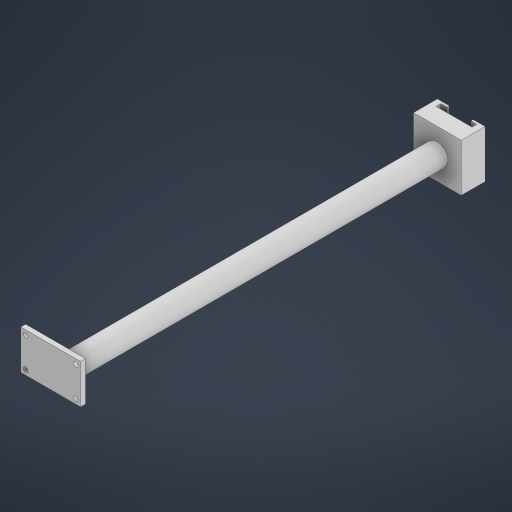
# Autodesk Inventor part: camera arm v1
Saved by Autodesk Inventor 2024 (Build 280153000, 153)
## iProperties
Created: 2023-06-18
Part Number: camera arm v1
Material: 일반
Document SubType Name: Modeling
Designer: 6gioc
Density: 1 g/cm^3
Appearance: 기본값
Author: 6gioc
## iProperties of the stored document camera arm v1_3D 인쇄.ipt
Created: 2023-06-20
Part Number: camera arm v1_3D 인쇄
Material: 일반
Document SubType Name: Modeling
Designer: 6gioc
Density: 1 g/cm^3
Appearance: 기본값
Author: 6gioc
Autodesk Inventor part; units mm, degrees
ref_plane "YZ Plane" through (0, 0, 0) normal (1, 0, 0) x (0, 1, 0)
ref_plane "XZ Plane" through (0, 0, 0) normal (0, 1, 0) x (-1, 0, 0)
ref_plane "XY Plane" through (0, 0, 0) normal (0, 0, 1) x (1, 0, 0)
sketch "스케치1" plane through (0, 0, 0) normal (0, 0, 1) x (1, 0, 0)
  line L0 (0, 0) -> (25, 0)
  line L1 (25, 0) -> (25, 16.5)
  line L2 (25, 16.5) -> (0, 16.5)
  line L3 (0, 16.5) -> (0, 0)
  circle A0 centre (23, 14.5) radius 1
  circle A1 centre (2, 14.5) radius 1
  circle A2 centre (2, 2) radius 1
  circle A3 centre (23, 2) radius 1
  circle A4 centre (12.5, 4.5) radius 4.5
  dimension "d0" = 25
  dimension "d1" = 16.5
  dimension "d2" = 2
  dimension "d3" = 2
  dimension "d4" = 2
  dimension "d5" = 2
  dimension "d6" = 2
  dimension "d7" = 2
  dimension "d8" = 2
  dimension "d9" = 2
  dimension "d10" = 2
  dimension "d11" = 2
  dimension "d12" = 2
  dimension "d13" = 2
  dimension "d14" = 12.5
  dimension "d15" = 12.5
  dimension "d18" = 9
  dimension "d19" = 12
  dimension "d20" = 16.5
  constraints: 8 end point, 5 centre point, 2 parallel, 1 horizontal, 1 perpendicular
  measures "d0" distance of L2.end L1.end
  measures "d1" distance of L1.end L0.end
  measures "d2" diameter of A0
  measures "d3" diameter of A1
  measures "d4" diameter of A2
  measures "d5" diameter of A3
  measures "d6" distance from line of L1 A0.centre
  measures "d7" distance from line of A0.centre L2
  measures "d8" distance from line of L1 A3.centre
  measures "d9" distance from line of L0 A3.centre
  measures "d10" distance from line of L0 A2.centre
  measures "d11" distance from line of L3 A2.centre
  measures "d12" distance from line of L3 A1.centre
  measures "d13" distance from line of A1.centre L2
  measures "d14" distance of A3.centre A0.centre
  measures "d15" distance of A2.centre A1.centre
  measures "d18" diameter of A4
  measures "d19" distance from line of A4.centre L2
  measures "d20" distance between parallel lines of L0 L2
extrude "돌출1" add sketch "스케치1" along normal blind 2 contours A4 | L3 L2 L1 L0
extrude "돌출2" add sketch "스케치1" against normal blind 160 contours A4
sketch "스케치2" plane through (12.5, 4.5, -160) normal (0, 0, -1) x (-1, 0, 0)
  line L0 (0, 0) -> (10, 0)
  line L1 (10, 0) -> (10, -10)
  line L2 (10, -10) -> (0, -10)
  line L3 (0, -10) -> (0, 0)
  line L4 (10, -10) -> (-10, -10)
  line L5 (-10, -10) -> (-10, 10)
  line L6 (-10, 10) -> (10, 10)
  line L7 (10, 10) -> (10, -10)
  point P0 (12.5, -4.5)
  dimension "d23" = 10
  dimension "d24" = 10
  dimension "d25" = 20
  dimension "d26" = 20
  constraints: 16 end point, 4 parallel, 2 horizontal, 2 perpendicular
  measures "d23" distance of L1.end L2.end
  measures "d24" distance of L0.end L1.end
  measures "d25" distance of L5.end L6.end
  measures "d26" distance of L4.end L5.end
extrude "돌출3" add sketch "스케치2" along normal blind 10
sketch "스케치3" plane through (2.5, -5.5, -160) normal (-1, 0, 0) x (0, 0, 1)
  line L0 (-10, 20) -> (-10, 0) projected
  line L1 (0, 20) -> (0, 0) projected
  line L2 (-10, 20) -> (0, 0)
  line L3 (-10, 0) -> (0, 20)
  circle A0 centre (-5, 10) radius 2.5
  line L4 (-5, 12.5) -> (-3.75, 12.1651)
  line L5 (-3.75, 12.1651) -> (-2.8349, 11.25)
  line L6 (-2.8349, 11.25) -> (-2.5, 10)
  line L7 (-2.5, 10) -> (-2.8349, 8.75)
  line L8 (-2.8349, 8.75) -> (-3.75, 7.8349)
  line L9 (-3.75, 7.8349) -> (-5, 7.5)
  line L10 (-5, 7.5) -> (-6.25, 7.8349)
  line L11 (-6.25, 7.8349) -> (-7.1651, 8.75)
  line L12 (-7.1651, 8.75) -> (-7.5, 10)
  line L13 (-7.5, 10) -> (-7.1651, 11.25)
  line L14 (-7.1651, 11.25) -> (-6.25, 12.1651)
  line L15 (-6.25, 12.1651) -> (-5, 12.5)
  point P0 (160, 5.5)
  dimension "d29" = 5
  constraints: 28 end point, 1 coincident, 1 midpoint, 1 vertical alignment, 27 other
extrude "돌출4" cut sketch "스케치3" against normal blind 15 contours L15 L4 L3 L2 | L2 L3 L10 L11 L12 L13 L14 L15 | L3 L2 L9 L10 | L3 L4 L5 L6 L7 L8 L9 L2
sketch "스케치4" plane through (2.5, 14.5, -160) normal (0, 1, 0) x (1, 0, 0)
  line L0 (17.5, 9) -> (2.5, 9)
  line L1 (2.5, 9) -> (2.5, 7)
  line L2 (2.5, 7) -> (17.5, 7)
  line L3 (17.5, 7) -> (17.5, 9)
  line L4 (0, 10) -> (20, 10) projected
  line L5 (20, 0) -> (20, 10) projected
  line L6 (15, 9) -> (5, 9)
  line L7 (5, 9) -> (5, 10)
  line L8 (5, 10) -> (15, 10)
  line L9 (15, 10) -> (15, 9)
  point P0 (-2.5, -160)
  point P1 (15, 9.5)
  point P2 (15, 10)
  point P3 (5, 9)
  dimension "d32" = 15
  dimension "d33" = 2
  dimension "d34" = 1
  dimension "d35" = 2.5
  dimension "d36" = 10
  dimension "d37" = 1
  dimension "d38" = 2.5
  constraints: 16 end point, 4 parallel, 2 horizontal, 2 perpendicular, 1 midpoint, 1 point on line
  measures "d32" distance of L2.end L1.end
  measures "d33" distance of L1.end L0.end
  measures "d34" distance between parallel lines of L4 L0
  measures "d35" distance between parallel lines of L5 L3
  measures "d36" distance of L7.end L8.end
  measures "d37" distance of L6.end L7.end
  measures "d38" distance from line of point (15, 9.5) L3
extrude "돌출5" cut sketch "스케치4" against normal blind 5
